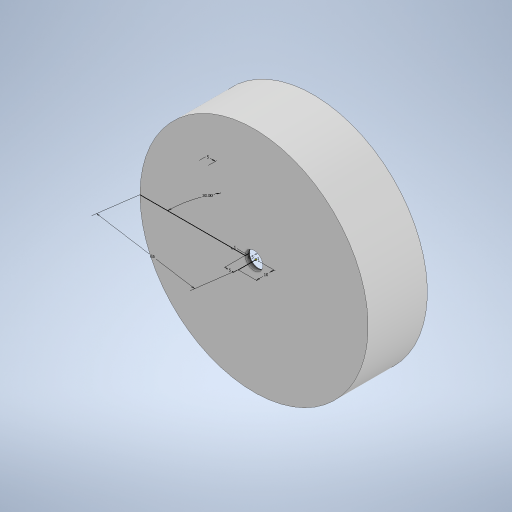
# Autodesk Inventor part: outterEdge
Saved by Autodesk Inventor 2023 (Build 270158000, 158)
## iProperties
Created: 2023-04-08
Part Number: outterEdge
Material: Generic
Document SubType Name: Modeling
Designer: lidang
Density: 1 g/cm^3
Appearance: Default
Author: lidang
Autodesk Inventor part; units mm, degrees
ref_plane "YZ Plane" through (0, 0, 0) normal (1, 0, 0) x (0, 1, 0)
ref_plane "XZ Plane" through (0, 0, 0) normal (0, 1, 0) x (-1, 0, 0)
ref_plane "XY Plane" through (0, 0, 0) normal (0, 0, 1) x (1, 0, 0)
sketch "Sketch1" plane through (0, 0, 0) normal (0, 1, 0) x (-1, 0, 0)
  line L0 (5, -1) -> (59.3739, -32.3928)
  line L1 (59.3739, -32.3928) -> (64.3739, -32.3928)
  line L2 (64.3739, -32.3928) -> (64.3739, 1)
  line L3 (64.3739, 1) -> (5, 1)
  line L4 (0, 10) -> (0, 0)
  line L5 (5, 1) -> (5, -1)
  line L6 (5, -1) -> (5, -1.5)
  line L7 (5, -1.5) -> (59.1574, -32.7678)
  line L8 (59.1574, -32.7678) -> (59.3739, -32.3928)
  dimension "d0" = 65
  dimension "d1" = 0
  dimension "d2" = 10
  dimension "d3" = 5
  dimension "d4" = 30
  dimension "d5" = 5
  dimension "d6" = 0.5
  dimension "d13" = 1
  dimension "d14" = 1
  constraints: 18 end point, 4 perpendicular, 1 horizontal, 1 parallel, 1 vertical
  measures "d0" distance of L2.end L4.start
  measures "d1" distance of point (0, 0) L4.end
  measures "d2" distance of L4.start L4.end
  measures "d3" distance of L0.end L1.end
  measures "d4" angle of L3 L0
  measures "d5" distance between parallel lines of L4 L5
  measures "d6" distance of L0.start L6.end
  measures "d13" vertical distance of point (0, 0) L0.start
  measures "d14" distance from line of point (0, 0) L3
revolve "Revolution1" add sketch "Sketch1" angle 360 about axis through (0, 0, 10) along (0, 0, -1) contours L5 L3 L2 L1 L0
extrude "Extrusion1" add sketch "Sketch1" along normal mid plane 2 contours L0 L8 L7 L6
pattern_circular "Circular Pattern1" count 70 over 360 about axis through (0, 0, 0) along (0, 0, -1) of "Extrusion1"
body "Solid1"
